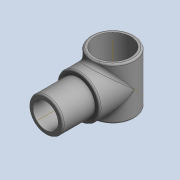
# Autodesk Inventor part: L114-7
Saved by Autodesk Inventor 2021 (Build 250183000, 183)
## iProperties
Created: 2020-04-23
Part Number: L114-7
Material: Generic
Document SubType Name: Modeling
Designer: Hannah
Density: 2.78424 g/cm^3
Appearance: Default
Mass: 270 g
Surface Area: 339.065 cm^2
Volume: 96.9745 cm^3
Author: Hannah
Autodesk Inventor part; units mm, degrees
ref_plane "YZ Plane" through (0, 0, 0) normal (1, 0, 0) x (0, 1, 0)
ref_plane "XZ Plane" through (0, 0, 0) normal (0, 1, 0) x (-1, 0, 0)
ref_plane "XY Plane" through (0, 0, 0) normal (0, 0, 1) x (1, 0, 0)
sketch "Sketch1" plane through (0, 0, 0) normal (0, 0, 1) x (1, 0, 0)
  circle A0 centre (0, 0) radius 21
  circle A1 centre (0, 0) radius 26.5
  circle A2 centre (0, 0) radius 15.5
  dimension "d1" = 53
  dimension "d2" = 42
  dimension "d34" = 31
  constraints: 3 centre point, 3 coincident
  measures "d1" diameter of A1
  measures "d2" diameter of A0
  measures "d34" diameter of A2
extrude "Extrusion1" add sketch "Sketch1" along normal blind 43 contours A0 | A1 | A2
sketch "Sketch2" plane through (0, 0, 0) normal (0, 1, 0) x (-1, 0, 0)
  circle A0 centre (0, 0) radius 22
  circle A1 centre (0, 0) radius 26.5
  dimension "d5" = 44
  dimension "d6" = 53
  constraints: 2 centre point, 2 coincident
  measures "d5" diameter of A0
  measures "d6" diameter of A1
extrude "Extrusion2" add sketch "Sketch2" along normal mid plane 64 contours A0 | A1
extrude "Extrusion4" add sketch "Sketch1" along normal blind 40 from surface at 43 contours A0 | A2
extrude "Extrusion3" cut sketch "Sketch2" against normal up to surface (64 mm away) from surface at 32 contours A0
extrude "Extrusion5" cut sketch "Sketch1" along normal through all contours A2
fillet "Fillet1" radius 5 2 edges at (0, 26.5, 26.5) (0, -26.5, 26.5)
hole "Hole1" at (0, 0, 0) direction (-1, 0, 0) diameter 8.376 end through all thread size "M10x1.5" class "6H" standard "ISO Metric profile"
fillet "Fillet2" radius 2 4 edges at (26.5, 32, 0) (26.5, -32, 0) (-21, 0, 83) (-26.5, 0, 43)
equation "\"d34\" = 2 * d2 - d1"
equation "\"d6\" = d1"
body "Solid1"
